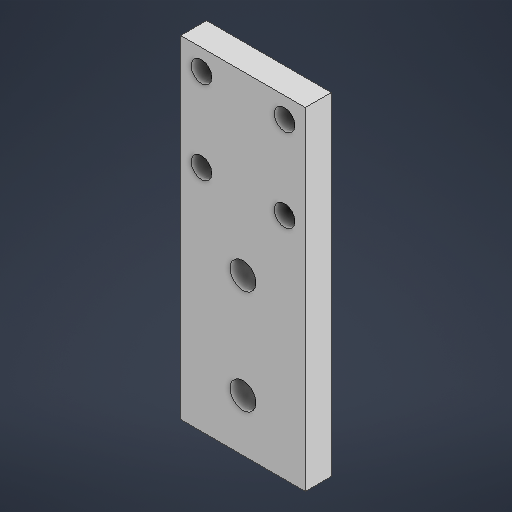
# Autodesk Inventor part: 2020 goRail Bracket
Saved by Autodesk Inventor 2026 (Build 300175050, 175E)
## iProperties
Created: 2025-11-14
Part Number: 2020 goRail Bracket
Material: Generic
Document SubType Name: Modeling
Designer: habbo
Density: 1 g/cm^3
Appearance: Default
Author: habbo
Autodesk Inventor part; units mm, degrees
ref_plane "YZ Plane" through (0, 0, 0) normal (1, 0, 0) x (0, 1, 0)
ref_plane "XZ Plane" through (0, 0, 0) normal (0, 1, 0) x (-1, 0, 0)
ref_plane "XY Plane" through (0, 0, 0) normal (0, 0, 1) x (1, 0, 0)
sketch "Sketch1" plane through (0, 0, 0) normal (0, 0, 1) x (1, 0, 0)
  line L0 (-12, -32) -> (12, -32)
  line L1 (12, -32) -> (12, 32)
  line L2 (12, 32) -> (-12, 32)
  line L3 (-12, 32) -> (-12, -32)
  line L4 (-12, -32) -> (12, 32) construction
  line L5 (12, -32) -> (-12, 32) construction
  circle A0 centre (-8, 28) radius 2
  circle A1 centre (-8, 12) radius 2
  circle A2 centre (8, 28) radius 2
  circle A3 centre (8, 12) radius 2
  circle A4 centre (0, -22) radius 2.5
  circle A5 centre (0, -2) radius 2.5
  point P0 (0, 0)
  dimension "d0" = 24
  dimension "d1" = 64
  dimension "d2" = 4
  dimension "d3" = 4
  dimension "d4" = 4
  dimension "d5" = 4
  dimension "d6" = 4
  dimension "d7" = 4
  dimension "d8" = 4
  dimension "d9" = 16
  dimension "d10" = 5
  dimension "d11" = 5
  dimension "d12" = 10
  dimension "d13" = 20
  dimension "d14" = 12
  constraints: 12 end point, 6 centre point, 3 vertical alignment, 2 horizontal alignment, 2 midpoint, 2 parallel, 1 horizontal, 1 perpendicular
  measures "d0" distance of L2.end L1.end
  measures "d1" distance of L1.end L0.end
  measures "d2" diameter of A0
  measures "d3" diameter of A1
  measures "d4" diameter of A2
  measures "d5" diameter of A3
  measures "d6" distance from line of L3 A0.centre
  measures "d7" distance from line of L2 A0.centre
  measures "d8" distance from line of A2.centre L1
  measures "d9" distance of A1.centre A0.centre
  measures "d10" diameter of A4
  measures "d11" diameter of A5
  measures "d12" distance from line of L0 A4.centre
  measures "d13" distance of A5.centre A4.centre
  measures "d14" distance from line of A5.centre L3
extrude "Extrusion1" add sketch "Sketch1" along normal mid plane 5
body "Solid1"
